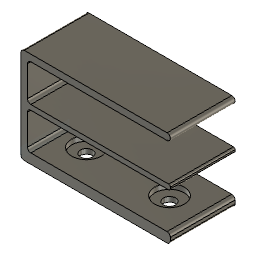
laptopMount (Autodesk Fusion 360 design; units mm, degrees)
part number: 2026-08-10-19-56-16-923
Autodesk Fusion 360 part; units mm, degrees
sketch "Sketch1" plane through (0, 0, 0) normal (0, 0, 1) x (1, 0, 0)
  line L0 (-28, 37) -> (62, 37)
  line L1 (62, 37) -> (62, 18)
  line L2 (62, 18) -> (-28, 18)
  line L3 (-28, 18) -> (-28, 37)
  dimension "d1" = 90
  dimension "d2" = 19
  constraint horizontal L0
  constraint vertical L1
  constraint horizontal L2
  constraint vertical L3
  measures "d1" distance of L0.start L0.end
  measures "d2" distance of L0.start L2.end
extrude "Extrude1" add sketch "Sketch1" along normal blind 6
sketch "Sketch2" plane through (0, 0, 6) normal (0, 0, 1) x (-1, 0, 0)
  line L0 (28, -37) -> (28, -18)
  line L1 (28, -18) -> (-62, -18)
  line L2 (-62, -18) -> (-62, -37)
  line L3 (-62, -37) -> (28, -37)
ref_plane "WorkPlane1" through (17, 27.5, 6) normal (0, 0, 1) x (-1, 0, 0)
sketch "Sketch3" plane through (0, 0, 6) normal (0, 0, 1) x (1, 0, 0)
  line L0 (17, 37) -> (17, 18)
  circle A0 centre (-8, 27.5) radius 8.9
  circle A1 centre (42, 27.5) radius 8.9
  circle A2 centre (-8, 27.5) radius 3.65
  circle A3 centre (42, 27.5) radius 3.65
  dimension "d13" = 17.8
  dimension "d14" = 17.8
  dimension "d15" = 7.3
  dimension "d16" = 7.3
  constraint vertical L0
  constraint concentric A0 A2
  constraint concentric A1 A3
  measures "d13" diameter of A0
  measures "d14" diameter of A1
  measures "d15" diameter of A2
  measures "d16" diameter of A3
extrude "Extrude2" cut sketch "Sketch3" against normal blind 7 contours A2 | A3
extrude "Extrude3" cut sketch "Sketch3" against normal blind 3
sketch "Sketch7" plane through (0, 0, 0) normal (0, 0, -1) x (1, 0, 0)
  circle A0 centre (42, -27.5) radius 3.65
  circle A1 centre (-8, -27.5) radius 3.65
  line L0 (62, -18) -> (-28, -18)
  line L1 (-28, -18) -> (-28, -37)
  line L2 (-28, -37) -> (62, -37)
  line L3 (62, -37) -> (62, -18)
  line L4 (-28, -18) -> (62, -18)
  line L5 (62, -18) -> (62, -8)
  line L6 (62, -8) -> (-28, -8)
  line L7 (-28, -8) -> (-28, -18)
  dimension "d37" = 10
  dimension "d38" = 90
  constraint horizontal L4
  constraint vertical L5
  constraint horizontal L6
  constraint vertical L7
  constraint coincident L0.end L1.start
  measures "d37" distance of L0.end L6.end
  measures "d38" distance of L0.end L0.start
extrude "Extrude7" add sketch "Sketch7" against normal blind 6 contours L0 L4 L5 L6 L7
sketch "Sketch8" plane through (-28, 0, 0) normal (-1, 0, 0) x (0, -1, 0)
  line L0 (-37, 0) -> (-8, 0)
  line L1 (-8, 0) -> (-8, 6)
  line L2 (-8, 6) -> (-37, 6)
  line L3 (-37, 6) -> (-37, 0)
ref_plane "WorkPlane3" through (17, 22.5, 0) normal (0, 0, -1) x (-1, 0, 0)
sketch "Sketch9" plane through (0, 0, 0) normal (0, 0, -1) x (-1, 0, 0)
  line L0 (-62, 37) -> (28, 37)
  line L1 (28, 37) -> (28, 47)
  line L2 (28, 47) -> (-62, 47)
  line L3 (-62, 47) -> (-62, 37)
  dimension "d42" = 90
  dimension "d43" = 10
  constraint horizontal L0
  constraint vertical L1
  constraint horizontal L2
  constraint vertical L3
  measures "d42" distance of L0.start L0.end
  measures "d43" distance of L0.start L2.end
extrude "Extrude8" add sketch "Sketch9" against normal blind 6
ref_plane "WorkPlane4" through (17, 8, 3) normal (0, -1, 0) x (1, 0, 0)
sketch "Sketch10" plane through (0, 8, 0) normal (0, -1, 0) x (-1, 0, 0)
  line L0 (28, -6) -> (24, -6)
  line L1 (24, -6) -> (24, -57.5)
  line L2 (24, -57.5) -> (28, -57.5)
  line L3 (28, -57.5) -> (28, -6)
  dimension "d47" = 4
  dimension "d48" = 51.5
  constraint horizontal L0
  constraint vertical L1
  constraint horizontal L2
  constraint vertical L3
  measures "d47" distance of L0.start L0.end
  measures "d48" distance of L0.start L2.end
extrude "Extrude9" add sketch "Sketch10" against normal blind 39
sketch "Sketch11" plane through (0, 8, 0) normal (0, -1, 0) x (1, 0, 0)
  line L0 (-28, 0) -> (62, 0)
  line L1 (62, 0) -> (62, 6)
  line L2 (62, 6) -> (-24, 6)
  line L3 (-24, 6) -> (-24, 57.5)
  line L4 (-24, 57.5) -> (-28, 57.5)
  line L5 (-28, 57.5) -> (-28, 0)
  line L6 (-28, 57.5) -> (62, 57.5)
  line L7 (62, 57.5) -> (62, 53.5)
  line L8 (62, 53.5) -> (-28, 53.5)
  line L9 (-28, 53.5) -> (-28, 57.5)
  dimension "d51" = 90
  dimension "d52" = 4
  constraint horizontal L6
  constraint vertical L7
  constraint horizontal L8
  constraint vertical L9
  constraint coincident L4.end L5.start
  measures "d51" distance of L4.end L6.end
  measures "d52" distance of L4.end L8.end
extrude "Extrude10" add sketch "Sketch11" against normal blind 39 contours L3 L6 L7 L8
sketch "Sketch12" plane through (0, 8, 0) normal (0, -1, 0) x (1, 0, 0)
  line L0 (-28, 0) -> (62, 0)
  line L1 (62, 0) -> (62, 6)
  line L2 (62, 6) -> (-24, 6)
  line L3 (-24, 6) -> (-24, 53.5)
  line L4 (-24, 53.5) -> (62, 53.5)
  line L5 (62, 53.5) -> (62, 57.5)
  line L6 (62, 57.5) -> (-28, 57.5)
  line L7 (-28, 57.5) -> (-28, 0)
  circle A0 centre (-24, 6) radius 22.25
  line L8 (-24, 28.25) -> (62, 28.25)
  line L9 (62, 28.25) -> (62, 31.25)
  line L10 (62, 31.25) -> (-24, 31.25)
  line L11 (-24, 31.25) -> (-24, 28.25)
  dimension "d55" = 44.5
  dimension "d56" = 86
  dimension "d57" = 3
  constraint coincident L2.end L3.start
  constraint horizontal L8
  constraint vertical L9
  constraint horizontal L10
  constraint vertical L11
  constraint coincident L3 L8.start
  constraint coincident A0 L8.start
  measures "d55" diameter of A0
  measures "d56" distance of L8.start L8.end
  measures "d57" distance of L8.start L10.end
extrude "Extrude11" add sketch "Sketch12" against normal blind 39 contours L3 L8 L9 L10 L11
fillet "Fillet3" radius 2 1 edges at (-28, 27.5, 57.5)
fillet "Fillet4" radius 2 1 edges at (-28, 27.5, 0)
fillet "Fillet5" radius 2 2 edges at (-24, 27.5, 53.5) (-24, 27.5, 28.25)
fillet "Fillet6" radius 2 2 edges at (-24, 27.5, 31.25) (-24, 27.5, 6)
fillet "Fillet7" radius 1 2 edges at (62, 27.5, 31.25) (62, 27.5, 28.25)
fillet "Fillet8" radius 2 4 edges at (62, 27.5, 57.5) (62, 27.5, 53.5) (62, 27.5, 6) (62, 27.5, 0)
